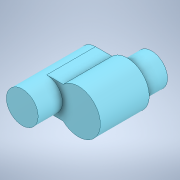
# Autodesk Inventor part: Component28
Saved by Autodesk Inventor 2022 (Build 260153000, 153)
## iProperties
Created: 2022-01-29
Part Number: Component28
Material: Generic
Document SubType Name: Modeling
Designer: Administrator
Density: 1 g/cm^3
Appearance: Default
Title: Component28
Author: Administrator
Autodesk Inventor part; units mm, degrees
ref_plane "YZ Plane" through (0, 0, 0) normal (1, 0, 0) x (0, 1, 0)
ref_plane "XZ Plane" through (0, 0, 0) normal (0, 1, 0) x (-1, 0, 0)
ref_plane "XY Plane" through (0, 0, 0) normal (0, 0, 1) x (1, 0, 0)
sketch "Sketch2" plane through (0, 0, 0) normal (0, 0, 1) x (1, 0, 0)
  line L0 (-6.9834, -3.25) -> (-3.5959, -3.25)
  arc A0 (-3.5959, -3.25) -> (-3.5959, 3.25) centre (-0.4834, 0) ccw
  circle A1 centre (-6.9834, 0) radius 3.25
  line L1 (7.6359, 0) -> (-9.8597, 0) construction
  line L2 (-6.9834, 3.25) -> (-3.5959, 3.25)
  circle A2 centre (-6.9834, 0) radius 3.25
  circle A3 centre (-0.4834, 0) radius 3.25
  point P0 (-7.0471, -3.1146)
  dimension "d6" = 6.5
  dimension "d7" = 9
  dimension "d8" = 6.5
  constraints: 6 end point, 3 horizontal, 2 centre point, 2 coincident, 2 point on circle, 2 point on line, 2 symmetric about line, 1 vertical alignment, 6 other
  measures "d7" diameter of A0
  measures "d8" distance of point (-6.983, 0) point (-0.483, 0)
extrude "Extrusion1" add sketch "Sketch2" along normal blind 10 contours A3 | A1 L2 A0 L0 | A1
extrude "Extrusion2" add sketch "Sketch2" against normal blind 5 contours A3
sketch "Sketch3" plane through (0, 0, 10) normal (0, 0, 1) x (1, 0, 0)
  arc A0 (-6.9834, 3.25) -> (-6.9834, -3.25) centre (-6.9834, 0) ccw projected
  line L0 (-3.5959, 3.25) -> (-6.9834, 3.25) projected
  arc A1 (-3.5959, -3.25) -> (-3.5959, 3.25) centre (-0.4834, 0) ccw
  line L1 (-6.9834, -3.25) -> (-3.5959, -3.25) projected
  circle A2 centre (-6.9834, 0) radius 3.25
  point P0 (-6.9834, -3.25)
  point P1 (-6.9834, 3.25)
  point P2 (-4.0488, -2.7456)
  point P3 (4.0134, -0.1685)
  dimension "d9" = 6.5
  constraints: 2 centre point, 2 point on circle
  measures "d9" diameter of A2
extrude "Extrusion3" add sketch "Sketch3" along normal blind 5 contours A2 A0
equation "\"d6\" = R"
equation "\"d7\" = R1"
equation "\"d8\" = R"
equation "\"d0\" = 2 * thickness"
equation "\"d2\" = thickness"
equation "\"d9\" = R"
equation "\"R\" = 6.5"
equation "\"thickness\" = 5"
equation "\"width\" = 6.5"
equation "\"R1\" = 9"
body "Solid1"
